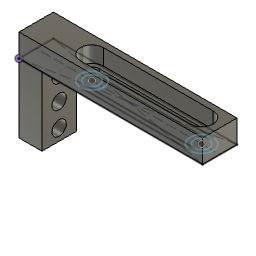
extender 3 v1 (Autodesk Fusion 360 design; units mm, degrees)
Autodesk Fusion 360 part; units mm, degrees
sketch "Sketch1" plane through (0, 0, 0) normal (0, 0, 1) x (1, 0, 0)
  line L0 (0, 0) -> (80, 0)
  line L1 (80, 0) -> (80, 15)
  line L2 (80, 15) -> (0, 15)
  line L3 (0, 15) -> (0, 0)
  line L4 (80, 15) -> (0, 0) construction
  line L5 (80, 0) -> (0, 15) construction
  line L6 (40, 7.5) -> (80, 7.5) construction
  line L7 (40, 7.5) -> (0, 7.5) construction
  circle A0 centre (72.075, 7.5) radius 5
  circle A1 centre (72.075, 7.5) radius 3.1375
  circle A2 centre (24.3001, 7.5) radius 5
  circle A3 centre (24.3001, 7.5) radius 3.1375
  line L8 (24.3001, 7.5) -> (24.3001, 15) construction
  line L9 (24.3001, 7.5) -> (24.3001, 0) construction
  line L10 (72.075, 7.5) -> (72.075, 15) construction
  line L11 (72.075, 7.5) -> (72.075, 0) construction
  line L12 (24.3001, 12.5) -> (72.075, 12.5)
  line L13 (24.3001, 2.5) -> (72.075, 2.5)
  line L14 (24.3001, 4.3625) -> (72.075, 4.3625)
  line L15 (24.3001, 10.6375) -> (72.075, 10.6375)
  dimension "d1" = 80
  dimension "d2" = 15
  dimension "d3" = 10
  dimension "d4" = 6.275
  dimension "d5" = 10
  dimension "d6" = 6.275
  constraint horizontal L0
  constraint vertical L1
  constraint horizontal L2
  constraint vertical L3
  constraint coincident L0.start L3.end
  constraint midpoint L4 L6.start
  constraint midpoint L1 L6.end
  constraint midpoint L3 L7.end
  constraint coincident L6 A0.centre
  constraint concentric A0 A1
  constraint coincident L7 A2.centre
  constraint concentric A2 A3
  constraint coincident A2.centre A3.centre
  constraint coincident L2 L8.end
  constraint perpendicular L2 L8
  constraint coincident L0 L9.end
  constraint perpendicular L0 L9
  constraint coincident A0.centre A1.centre
  constraint coincident L2 L10.end
  constraint perpendicular L2 L10
  constraint coincident L0 L11.end
  constraint perpendicular L0 L11
  constraint coincident A2 L12.start
  constraint coincident L8 L12.start
  constraint coincident A0 L12.end
  constraint coincident L10 L12.end
  constraint coincident A2 L13.start
  constraint coincident L9 L13.start
  constraint coincident A0 L13.end
  constraint coincident L11 L13.end
  constraint tangent A0 L13
  constraint coincident A3 L14.start
  constraint coincident L9 L14.start
  constraint coincident A1 L14.end
  constraint coincident L11 L14.end
  constraint coincident A3 L15.start
  constraint coincident L8 L15.start
  constraint coincident A1 L15.end
  constraint coincident L10 L15.end
  measures "d1" distance of L0.start L0.end
  measures "d2" distance of L0.start L2.end
  measures "d3" diameter of A0
  measures "d4" diameter of A1
  measures "d5" diameter of A2
  measures "d6" diameter of A3
extrude "Extrude1" add sketch "Sketch1" along normal blind 10 makes body 1
extrude "Extrude2" add sketch "Sketch1" along normal blind 3 separate body contours A0 A1 L14 L15 | A0 A2 L12 L15 | A0 A2 L13 L14 | A2 A3 L14 L15 picked at (71.828, 11.8608) picked at (21.1521, 10.5276) makes body 2
sketch "Sketch2" plane through (0, 0, 0) normal (0, 0, 1) x (1, 0, 0)
  line L0 (0, 0) -> (10, 0)
  line L1 (10, 0) -> (10, 15)
  line L2 (10, 15) -> (0, 15)
  line L3 (0, 15) -> (0, 0)
  dimension "d11" = 10
  dimension "d12" = 15
  constraint horizontal L0
  constraint vertical L1
  constraint horizontal L2
  constraint vertical L3
  constraint coincident L0.start L3.end
  measures "d11" distance of L0.start L0.end
  measures "d12" distance of L0.start L2.end
extrude "Extrude3" add sketch "Sketch2" against normal blind 30 bodies 1
sketch "Sketch3" plane through (0, 0, 0) normal (-1, 0, 0) x (0, -1, 0)
  line L0 (0, -30) -> (0, 10)
  line L1 (0, 10) -> (-15, 10)
  line L2 (-15, 10) -> (-15, -30)
  line L3 (-15, -30) -> (0, -30)
  line L4 (-15, -30) -> (0, 0) construction
  line L5 (-15, 0) -> (0, -30) construction
  line L6 (-15, -10) -> (0, -10) construction
  line L7 (-15, -20) -> (0, -20) construction
  line L8 (-7.5, -15) -> (-7.5, 10) construction
  line L9 (-7.5, -15) -> (-7.5, -30) construction
  line L10 (-15, -20) -> (0, -30) construction
  line L11 (-15, -30) -> (0, -20) construction
  line L12 (0, -20) -> (-15, -10) construction
  line L13 (-15, -20) -> (0, -10) construction
  line L14 (0, -10) -> (-15, 0) construction
  line L15 (-15, -10) -> (0, 0) construction
  circle A0 centre (-7.5, -5) radius 3.1375
  circle A1 centre (-7.5, -15) radius 3.1375
  circle A2 centre (-7.5, -25) radius 3.1375
  dimension "d15" = 10
  dimension "d16" = 20
  dimension "d17" = 6.275
  dimension "d18" = 6.275
  dimension "d19" = 6.275
  constraint coincident L2.end L3.start
  constraint coincident L4.end L15.end
  constraint coincident L2 L5.start
  constraint coincident L0.start L3.end
  constraint midpoint L2 L6.start
  constraint midpoint L0 L6.end
  constraint coincident L2 L7.start
  constraint perpendicular L2 L7
  constraint midpoint L5 L8.start
  constraint midpoint L1 L8.end
  constraint midpoint L3 L9.end
  constraint parallel L10 L12
  constraint parallel L12 L14
  constraint midpoint L15 A0.centre
  constraint coincident L8.start L9.start
  constraint midpoint L11 A2.centre
  measures "d15" distance of L3 L7
  measures "d16" distance of L3 L6
  measures "d17" diameter of A0
  measures "d18" diameter of A1
  measures "d19" diameter of A2
extrude "Extrude4" cut sketch "Sketch3" against normal blind 11 contours A0 | A1 | A2 bodies 1
